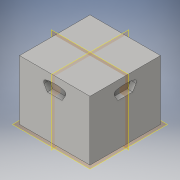
# Autodesk Inventor part: POWER CUBE
Saved by Autodesk Inventor 2016 SP2 (Build 200236200, 236)
## iProperties
Created: 2018-01-09
Part Number: POWER CUBE
Material: Generic
Document SubType Name: Modeling
Designer: CAD
Density: 1 g/cm^3
Appearance: Default
Author: CAD
Autodesk Inventor part; units mm, degrees
sketch "Sketch1" plane through (0, 0, 0) normal (0, 1, 0) x (-1, 0, 0)
  line L0 (165.1, 165.1) -> (-165.1, 165.1)
  line L1 (-165.1, 165.1) -> (-165.1, -165.1)
  line L2 (-165.1, -165.1) -> (165.1, -165.1)
  line L3 (165.1, -165.1) -> (165.1, 165.1)
  point P0 (0, 0)
  dimension "d0" = 330.2
  dimension "d1" = 330.2
  dimension "d2" = 165.1
  dimension "d3" = 165.1
  constraints: 8 end point, 2 parallel, 1 horizontal, 1 perpendicular
  measures "d0" distance of L2.end L1.end
  measures "d1" distance of L2.end L0.start
  measures "d2" distance from line of point (0, 0) L3
  measures "d3" distance from line of point (0, 0) L2
extrude "Extrusion1" add sketch "Sketch1" along normal blind 279.4
sketch "Sketch2" plane through (-165.1, 0, 165.1) normal (0, 0, 1) x (1, 0, 0)
  line L0 (0, 279.4) -> (330.2, 279.4) projected
  line L1 (165.1, 279.4) -> (165.1, 247.65)
  arc A0 (207.6282, 242.4889) -> (122.5718, 242.4889) centre (165.1, 69.85) ccw
  line L2 (130.175, 196.85) -> (200.025, 196.85)
  line L3 (200.025, 196.85) -> (215.589, 223.8076)
  line L4 (130.175, 196.85) -> (114.611, 223.8076)
  arc A1 (122.5718, 242.4889) -> (114.611, 223.8076) centre (125.6096, 230.1576) ccw
  arc A2 (215.589, 223.8076) -> (207.6282, 242.4889) centre (204.5904, 230.1576) ccw
  point P0 (165.1, 0)
  dimension "d6" = 31.75
  dimension "d8" = 177.8
  dimension "d10" = 0
  dimension "d11" = 69.85
  dimension "d12" = 34.925
  dimension "d13" = 50.8
  dimension "d16" = 120
  dimension "d17" = 120
  dimension "d18" = 12.7
  constraints: 8 end point, 7 point on circle, 4 tangent, 3 centre point, 1 equal radius, 1 horizontal, 1 midpoint, 1 vertical
  measures "d6" distance of L1.start L1.end
  measures "d8" radius of A0
  measures "d10" distance from line of L1 A0.centre
  measures "d11" distance of L2.start L2.end
  measures "d12" distance from line of L1 L2.end
  measures "d13" distance from line of L1.end L2
  measures "d16" angle of L2 L4
  measures "d17" angle of L2 L3
  measures "d18" radius of A1
extrude "Extrusion2" cut sketch "Sketch2" against normal blind 25.4
sketch "Sketch3" plane through (165.1, 0, 165.1) normal (1, 0, 0) x (0, 0, -1)
  arc A0 (207.6282, 242.4889) -> (122.5718, 242.4889) centre (165.1, 69.85) ccw
  line L0 (130.175, 196.85) -> (200.025, 196.85)
  line L1 (200.025, 196.85) -> (215.589, 223.8076)
  line L2 (130.175, 196.85) -> (114.611, 223.8076)
  arc A1 (122.5718, 242.4889) -> (114.611, 223.8076) centre (125.6096, 230.1576) ccw
  arc A2 (215.589, 223.8076) -> (207.6282, 242.4889) centre (204.5904, 230.1576) ccw
  line L3 (0, 279.4) -> (330.2, 279.4) projected
  point P0 (165.1, 0)
  point P1 (165.1, 247.65)
  dimension "d21" = 177.8
  dimension "d22" = 69.85
  dimension "d23" = 50.8
  dimension "d24" = 120
  dimension "d25" = 120
  dimension "d26" = 12.7
  dimension "d27" = 31.75
  dimension "d28" = 34.925
  constraints: 7 point on circle, 6 end point, 4 tangent, 3 centre point, 1 equal radius, 1 horizontal
  measures "d21" radius of A0
  measures "d22" distance of L0.start L0.end
  measures "d23" distance from line of point (165.1, 247.65) L0
  measures "d24" angle of L0 L2
  measures "d25" angle of L0 L1
  measures "d26" radius of A1
  measures "d27" distance from line of L3 point (165.1, 247.65)
  measures "d28" horizontal distance of point (165.1, 0) L0.end
extrude "Extrusion3" cut sketch "Sketch3" against normal blind 25.4
mirror "Mirror1" about plane through (0, 0, 0) normal (0, 0, 1) of "Extrusion2"
mirror "Mirror2" about plane through (0, 0, 0) normal (1, 0, 0) of "Extrusion3"
equation "\"d12\" = 0.5 * d11"
body "Solid1"
